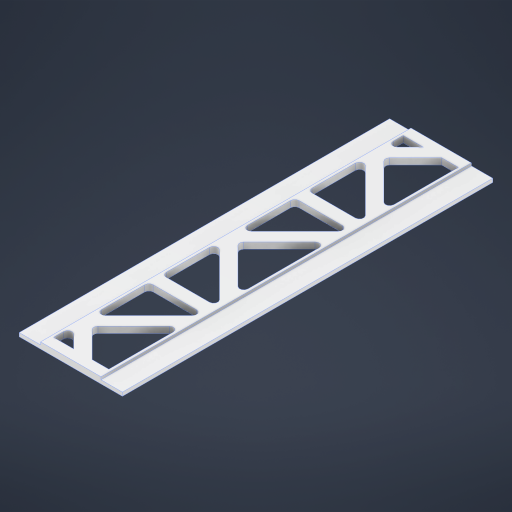
# Autodesk Inventor part: BackYflanec
Saved by Autodesk Inventor 2024 (Build 280153000, 153)
## iProperties
Created: 2023-01-15
Part Number: BackYflanec
Material: Aluminum 6061
Document SubType Name: Modeling
Designer: KirikDK
Density: 2.7 g/cm^3
Appearance: Aluminum - Flat
Mass: 2260.71 g
Surface Area: 2409.27 cm^2
Volume: 837.3 cm^3
Author: KirikDK
Autodesk Inventor part; units mm, degrees
ref_plane "YZ Plane" through (0, 0, 0) normal (1, 0, 0) x (0, 1, 0)
ref_plane "XZ Plane" through (0, 0, 0) normal (0, 1, 0) x (-1, 0, 0)
ref_plane "XY Plane" through (0, 0, 0) normal (0, 0, 1) x (1, 0, 0)
sketch "Эскиз1" plane through (0, 0, 0) normal (0, 1, 0) x (-1, 0, 0)
  line L0 (131.25, 393.75) -> (-8.75, 393.75)
  line L1 (-8.75, 393.75) -> (-8.75, -383.25)
  line L2 (-8.75, -383.25) -> (131.25, -383.25)
  line L3 (131.25, -383.25) -> (131.25, 393.75)
  point P0 (0, 0)
  dimension "d0" = 777
  dimension "d1" = 140
  constraints: 8 end point, 2 parallel, 1 horizontal, 1 perpendicular
  measures "d0" distance of L2.end L0.start
  measures "d1" distance of L0.start L0.end
sketch "Эскиз1 outline for Выдавливание1" plane through (0, 0, 0) normal (0, 1, 0) x (-1, 0, 0)
  line L0 (131.25, -383.25) -> (131.25, 393.75)
  line L1 (-8.75, -383.25) -> (131.25, -383.25)
  line L2 (-8.75, 393.75) -> (-8.75, -383.25)
  line L3 (131.25, 393.75) -> (-8.75, 393.75)
extrude "Выдавливание1" add sketch "Эскиз1 outline for Выдавливание1" along normal blind 12
sketch "Эскиз2" plane through (0, 12, 0) normal (0, 1, 0) x (1, 0, 0)
  line L0 (-146.25, -400) -> (-119.25, -400)
  line L1 (-119.25, -400) -> (-119.25, 402)
  line L2 (-119.25, 402) -> (-146.25, 402)
  line L3 (-146.25, 402) -> (-146.25, -400)
  line L4 (34.75, 391) -> (-3.25, 391)
  line L5 (-3.25, 391) -> (-3.25, -414)
  line L6 (-3.25, -414) -> (34.75, -414)
  line L7 (34.75, -414) -> (34.75, 391)
  line L8 (8.75, 383.25) -> (-131.25, 383.25) projected
  line L9 (-131.25, 383.25) -> (-131.25, -393.75) projected
  line L10 (-131.25, -393.75) -> (8.75, -393.75) projected
  line L11 (8.75, -393.75) -> (8.75, 383.25) projected
  point P0 (0, 0)
  point P1 (-3.25, 383.25)
  point P2 (-3.25, -393.75)
  point P3 (-119.25, -393.75)
  point P4 (-119.25, 383.25)
  dimension "d4" = 12
  dimension "d5" = 12
  constraints: 16 end point, 4 parallel, 2 horizontal, 2 perpendicular
  measures "d4" distance between parallel lines of L11 L5
  measures "d5" distance between parallel lines of L9 L1
sketch "Эскиз2 outline for Выдавливание2" plane through (0, 12, 0) normal (0, 1, 0) x (1, 0, 0)
  line L0 (8.75, -393.75) -> (8.75, 383.25)
  line L1 (-3.25, -393.75) -> (8.75, -393.75)
  line L2 (-3.25, 383.25) -> (-3.25, -393.75)
  line L3 (8.75, 383.25) -> (-3.25, 383.25)
  line L4 (-131.25, 383.25) -> (-131.25, -393.75)
  line L5 (-119.25, 383.25) -> (-131.25, 383.25)
  line L6 (-119.25, -393.75) -> (-119.25, 383.25)
  line L7 (-131.25, -393.75) -> (-119.25, -393.75)
extrude "Выдавливание2" cut sketch "Эскиз2 outline for Выдавливание2" against normal blind 5
sketch "Эскиз3" plane through (0, 12, 0) normal (0, 1, 0) x (1, 0, 0)
  line L0 (-3.25, -393.75) -> (-3.25, 383.25)
  line L1 (-3.25, 383.25) -> (-119.25, 383.25)
  line L2 (-119.25, 383.25) -> (-119.25, -393.75)
  line L3 (-119.25, -393.75) -> (-3.25, -393.75)
  line L4 (-114.25, -388.75) -> (-114.25, 378.25)
  line L5 (-114.25, 378.25) -> (-8.25, 378.25)
  line L6 (-8.25, 378.25) -> (-8.25, -388.75)
  line L7 (-8.25, -388.75) -> (-114.25, -388.75)
  line L8 (8.75, -393.75) -> (8.75, 383.25)
  line L9 (-131.25, 383.25) -> (-131.25, -393.75)
  line L10 (-131.25, -285.25) -> (8.75, -145.25)
  line L11 (8.75, -145.25) -> (-131.25, -5.25)
  line L12 (-131.25, -5.25) -> (8.75, 134.75)
  line L13 (8.75, 134.75) -> (-131.25, 274.75)
  line L14 (-131.25, 274.75) -> (-10.404914, 395.595086)
  line L15 (-131.25, 383.25) -> (-119.25, 383.25)
  line L16 (-131.25, -285.25) -> (119.241642, -535.741642)
  line L17 (35.67767, 406.32233) -> (-95.894661, 274.75)
  line L18 (-95.894661, 274.75) -> (44.105339, 134.75)
  line L19 (44.105339, 134.75) -> (-95.894661, -5.25)
  line L20 (-95.894661, -5.25) -> (44.105339, -145.25)
  line L21 (44.105339, -145.25) -> (-95.894661, -285.25)
  line L22 (-95.894661, -285.25) -> (136.919311, -518.063972)
  line L23 (-3.25, -393.75) -> (-3.25, 383.25)
  line L24 (-3.25, -173.25) -> (-3.25, -133.25)
  line L25 (-3.25, 142.75) -> (-3.25, 122.75)
  circle A0 centre (8.75, -145.25) radius 12.5
  circle A1 centre (8.75, 134.75) radius 12.5
  line L26 (8.75, 147.25) -> (-124, 147.25)
  line L27 (-124, 147.25) -> (-124, 122.25)
  line L28 (-124, 122.25) -> (8.75, 122.25)
  line L29 (8.75, 122.25) -> (8.75, 147.25)
  line L30 (8.75, -132.75) -> (-131.25, -132.75)
  line L31 (-131.25, -132.75) -> (-131.25, -157.75)
  line L32 (-131.25, -157.75) -> (8.75, -157.75)
  line L33 (8.75, -157.75) -> (8.75, -132.75)
  point P0 (0, 0)
  point P1 (-27.75, 378.25)
  point P2 (-114.25, 291.75)
  point P3 (-114.25, 257.75)
  point P4 (-8.25, 151.75)
  point P5 (-91.25, -0.605339)
  point P6 (-8.25, 82.394661)
  point P7 (-8.25, 187.105339)
  point P8 (-91.25, 270.105339)
  point P9 (-8.25, 117.75)
  point P10 (-114.25, 11.75)
  point P11 (-114.25, -22.25)
  point P12 (-8.25, -128.25)
  point P13 (-91.25, -280.605339)
  point P14 (-8.25, -197.605339)
  point P15 (-8.25, -92.894661)
  point P16 (-91.25, -9.894661)
  point P17 (-114.25, -302.25)
  point P18 (-27.75, -388.75)
  point P19 (-8.25, -162.25)
  point P20 (-114.25, -268.25)
  point P21 (-8.25, 362.394661)
  point P22 (-91.25, 279.394661)
  point P23 (-91.25, -289.894661)
  point P24 (-8.25, -372.894661)
  point P25 (-114.25, 147.25)
  point P26 (-8.25, 147.25)
  point P27 (-8.25, 122.25)
  point P28 (-114.25, 122.25)
  point P29 (-114.25, -132.75)
  point P30 (-8.25, -132.75)
  point P31 (-8.25, -157.75)
  point P32 (-114.25, -157.75)
  dimension "d34" = 25
  dimension "d35" = 25
  dimension "d8" = 5
  dimension "d11" = 90
  dimension "d12" = 90
  dimension "d13" = 90
  dimension "d15" = 90
  dimension "d16" = 90
  dimension "d17" = 108.5
  dimension "d18" = 45
  dimension "d22" = 25
  constraints: 52 end point, 9 point on line, 4 parallel, 2 coincident, 2 horizontal, 2 perpendicular, 2 vertical alignment, 1 midpoint, 12 other
  measures "d8" distance between parallel lines of L2 L4
  measures "d11" angle of L11 L10
  measures "d12" angle of L12 L11
  measures "d13" angle of L13 L12
  measures "d15" angle of L14 L13
  measures "d16" angle of L10 L16
  measures "d17" distance of L9.start L13.end
  measures "d18" angle of L8 L16
  measures "d22" distance between parallel lines of L20 L11
sketch "Эскиз3 outline for Выдавливание4" plane through (0, 12, 0) normal (0, 1, 0) x (1, 0, 0)
  line L0 (-95.894661, -285.25) -> (-8.25, -372.894661)
  line L1 (-8.25, -197.605339) -> (-95.894661, -285.25)
  line L2 (-8.25, -372.894661) -> (-8.25, -197.605339)
  line L3 (-95.894661, -5.25) -> (-8.25, -92.894661)
  line L4 (-8.25, 82.394661) -> (-95.894661, -5.25)
  line L5 (-8.25, -92.894661) -> (-8.25, 82.394661)
  line L6 (-95.894661, 274.75) -> (-8.25, 187.105339)
  line L7 (-8.25, 362.394661) -> (-95.894661, 274.75)
  line L8 (-8.25, 187.105339) -> (-8.25, 362.394661)
  line L9 (-114.25, 291.75) -> (-27.75, 378.25)
  line L10 (-114.25, 378.25) -> (-114.25, 291.75)
  line L11 (-27.75, 378.25) -> (-114.25, 378.25)
  line L12 (-27.75, -388.75) -> (-114.25, -302.25)
  line L13 (-114.25, -388.75) -> (-27.75, -388.75)
  line L14 (-114.25, -302.25) -> (-114.25, -388.75)
  line L15 (-114.25, 147.25) -> (-8.25, 147.25)
  line L16 (-114.25, 257.75) -> (-114.25, 147.25)
  line L17 (-8.25, 151.75) -> (-114.25, 257.75)
  line L18 (-8.25, 147.25) -> (-8.25, 151.75)
  line L19 (-8.25, 122.25) -> (-114.25, 122.25)
  line L20 (-8.25, 117.75) -> (-8.25, 122.25)
  line L21 (-114.25, 11.75) -> (-8.25, 117.75)
  line L22 (-114.25, 122.25) -> (-114.25, 11.75)
  line L23 (-114.25, -132.75) -> (-8.25, -132.75)
  line L24 (-114.25, -22.25) -> (-114.25, -132.75)
  line L25 (-8.25, -128.25) -> (-114.25, -22.25)
  line L26 (-8.25, -132.75) -> (-8.25, -128.25)
  line L27 (-8.25, -157.75) -> (-114.25, -157.75)
  line L28 (-8.25, -162.25) -> (-8.25, -157.75)
  line L29 (-114.25, -268.25) -> (-8.25, -162.25)
  line L30 (-114.25, -157.75) -> (-114.25, -268.25)
extrude "Выдавливание4" cut sketch "Эскиз3 outline for Выдавливание4" against normal blind 23
sketch "Sketch5" plane through (8.75, 0, -383.25) normal (0, 0, -1) x (-1, 0, 0)
  line L0 (0, 0) -> (0, 7) projected
  line L1 (0, 0) -> (-29, 0)
  line L2 (-29, 0) -> (-29, 7)
  line L3 (-29, 7) -> (0, 7)
  line L4 (0, 7) -> (0, 0)
  line L5 (140, 0) -> (140, 7) projected
  line L6 (140, 0) -> (169, 0)
  line L7 (169, 0) -> (169, 7)
  line L8 (169, 7) -> (140, 7)
  line L9 (140, 7) -> (140, 0)
  line L10 (128, 12) -> (128, 7) projected
  line L11 (12, 7) -> (12, 12) projected
  point P0 (8.75, 0)
  dimension "d41" = 41
  dimension "d42" = 41
  constraints: 16 end point, 4 parallel, 2 horizontal, 2 perpendicular
  measures "d41" distance between parallel lines of L10 L7
  measures "d42" distance between parallel lines of L11 L2
sketch "Sketch5 outline for Extrusion6" plane through (8.75, 0, -383.25) normal (0, 0, -1) x (-1, 0, 0)
  line L0 (169, 7) -> (140, 7)
  line L1 (169, 0) -> (169, 7)
  line L2 (140, 0) -> (169, 0)
  line L3 (140, 7) -> (140, 0)
  line L4 (0, 7) -> (-29, 7)
  line L5 (0, 0) -> (0, 7)
  line L6 (-29, 0) -> (0, 0)
  line L7 (-29, 7) -> (-29, 0)
extrude "Extrusion6" add sketch "Sketch5 outline for Extrusion6" against normal up to surface (777 mm away)
fillet "Fillet2" radius 8 31 edges at (-8.25, 6, -187.1053) (-8.25, 6, -147.25) (-8.25, 6, -117.75) (-8.25, 6, 92.8947) (-8.25, 6, 132.75) (-8.25, 6, 162.25) (-8.25, 6, 372.8947) (-27.75, 6, 388.75) (-27.75, 6, -378.25) (-8.25, 6, -362.3947) (-8.25, 6, -122.25) (-8.25, 6, -151.75) (-8.25, 6, -82.3947) (-8.25, 6, 128.25) (-8.25, 6, 157.75) (-8.25, 6, 197.6053) (-114.25, 6, -378.25) (-114.25, 6, -257.75) (-114.25, 6, -122.25) (-114.25, 6, 22.25) (-114.25, 6, 157.75) (-114.25, 6, 302.25) (-95.8947, 6, 5.25) (-95.8947, 6, 285.25) (-114.25, 6, 268.25) (-114.25, 6, -11.75) (-114.25, 6, -147.25) (-114.25, 6, -291.75) (-95.8947, 6, -274.75) (-114.25, 6, 132.75) (-114.25, 6, 388.75)
sketch "Sketch6" plane through (0, 7, 0) normal (0, 1, 0) x (1, 0, 0)
  line L0 (-160.25, 383.25) -> (-119.25, 383.25) projected
  line L1 (37.75, 383.25) -> (37.75, -393.75) projected
  line L2 (-160.25, 383.25) -> (37.75, 383.25)
  line L3 (37.75, 383.25) -> (37.75, 350.25)
  line L4 (37.75, 350.25) -> (-160.25, 350.25)
  line L5 (-160.25, 350.25) -> (-160.25, 383.25)
  line L6 (-160.25, -393.75) -> (37.75, -393.75) projected
  line L7 (-160.25, -393.75) -> (37.75, -393.75)
  line L8 (37.75, -393.75) -> (37.75, -360.75)
  line L9 (37.75, -360.75) -> (-160.25, -360.75)
  line L10 (-160.25, -360.75) -> (-160.25, -393.75)
  point P0 (0, 0)
  point P1 (37.75, -360.75)
  dimension "d43" = 33
  dimension "d44" = 33
  constraints: 16 end point, 4 parallel, 2 horizontal, 2 perpendicular, 2 point on line
  measures "d43" distance between parallel lines of L2 L4
  measures "d44" distance between parallel lines of L9 L6
sketch "Sketch6 outline for Extrusion7" plane through (0, 7, 0) normal (0, 1, 0) x (1, 0, 0)
  line L0 (-160.25, -360.75) -> (-160.25, -393.75)
  line L1 (37.75, -360.75) -> (-160.25, -360.75)
  line L2 (37.75, -393.75) -> (37.75, -360.75)
  line L3 (-160.25, -393.75) -> (37.75, -393.75)
  line L4 (-160.25, 383.25) -> (-160.25, 350.25)
  line L5 (-160.25, 350.25) -> (37.75, 350.25)
  line L6 (37.75, 350.25) -> (37.75, 383.25)
  line L7 (37.75, 383.25) -> (-160.25, 383.25)
extrude "Extrusion7" cut sketch "Sketch6 outline for Extrusion7" along normal mid plane 30
sketch "Sketch7" plane through (0, 12, 0) normal (0, 1, 0) x (1, 0, 0)
  line L0 (-3.25, -360.75) -> (-3.25, 350.25) projected
  line L1 (-119.25, -360.75) -> (-3.25, -360.75)
  line L2 (-3.25, -360.75) -> (-3.25, -340.75)
  line L3 (-3.25, -340.75) -> (-119.25, -340.75)
  line L4 (-119.25, -340.75) -> (-119.25, -360.75)
  line L5 (-119.25, 350.25) -> (-119.25, -360.75) projected
  line L6 (-3.25, 350.25) -> (-119.25, 350.25)
  line L7 (-119.25, 350.25) -> (-119.25, 330.25)
  line L8 (-119.25, 330.25) -> (-3.25, 330.25)
  line L9 (-3.25, 330.25) -> (-3.25, 350.25)
  point P0 (0, 0)
  point P1 (-3.25, 330.25)
  dimension "d47" = 20
  dimension "d48" = 20
  constraints: 16 end point, 4 parallel, 2 horizontal, 2 perpendicular, 2 point on line
  measures "d47" distance of L3.end L1.start
  measures "d48" distance between parallel lines of L6 L8
sketch "Sketch7 outline for Extrusion8" plane through (0, 12, 0) normal (0, 1, 0) x (1, 0, 0)
  line L0 (-119.25, -360.75) -> (-3.25, -360.75)
  line L1 (-119.25, -340.75) -> (-119.25, -360.75)
  line L2 (-3.25, -340.75) -> (-119.25, -340.75)
  line L3 (-3.25, -360.75) -> (-3.25, -340.75)
  line L4 (-3.25, 350.25) -> (-119.25, 350.25)
  line L5 (-3.25, 330.25) -> (-3.25, 350.25)
  line L6 (-119.25, 330.25) -> (-3.25, 330.25)
  line L7 (-119.25, 350.25) -> (-119.25, 330.25)
extrude "Extrusion8" add sketch "Sketch7 outline for Extrusion8" against normal up to surface (12 mm away)
